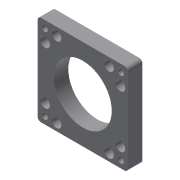
# Autodesk Inventor part: 20_IM_LED_holder
Saved by Autodesk Inventor 2019.4 (Build 234330000, 330)
## iProperties
Created: 2020-10-28
Part Number: 20_IM_LED_holder
Material: Generic
Document SubType Name: Modeling
Designer: wanghaoran
Density: 1 g/cm^3
Appearance: Default
Author: wanghaoran
Autodesk Inventor part; units mm, degrees
ref_plane "YZ Plane" through (0, 0, 0) normal (1, 0, 0) x (0, 1, 0)
ref_plane "XZ Plane" through (0, 0, 0) normal (0, 1, 0) x (-1, 0, 0)
ref_plane "XY Plane" through (0, 0, 0) normal (0, 0, 1) x (1, 0, 0)
sketch "Sketch1" plane through (0, 0, 0) normal (0, 0, 1) x (1, 0, 0)
  line L0 (-25, 25) -> (25, 25)
  line L1 (25, 25) -> (25, -25)
  line L2 (25, -25) -> (-25, -25)
  line L3 (-25, -25) -> (-25, 25)
  line L4 (-25, 25) -> (25, -25) construction
  line L5 (25, 25) -> (-25, -25) construction
  circle A0 centre (0, 0) radius 16
  circle A1 centre (-20.8, -14.5) radius 2.65
  circle A2 centre (-14.5, -20.8) radius 2.65
  circle A3 centre (-20.8, 14.5) radius 2.65
  circle A4 centre (20.8, -14.5) radius 2.65
  circle A5 centre (20.8, 14.5) radius 2.65
  circle A6 centre (-14.5, 20.8) radius 2.65
  circle A7 centre (14.5, -20.8) radius 2.65
  circle A8 centre (14.5, 20.8) radius 2.65
  dimension "d0" = 50
  dimension "d1" = 50
  dimension "d2" = 32
  dimension "d5" = 5.3
  dimension "d6" = 4.2
  dimension "d8" = 10.5
  dimension "d11" = 29
  dimension "d14" = 41.6
  constraints: 12 end point, 9 centre point, 4 symmetric about line, 2 horizontal, 2 midpoint, 2 parallel, 1 coincident, 1 perpendicular, 1 vertical, 10 other
  measures "d0" distance of L1.end L2.end
  measures "d1" distance of L0.end L1.end
  measures "d2" diameter of A0
  measures "d5" diameter of A1
  measures "d6" distance from line of A1.centre L3
  measures "d8" distance from line of L2 A1.centre
  measures "d11" distance of A1.centre A3.centre
  measures "d14" distance of A1.centre A4.centre
extrude "Extrusion1" add sketch "Sketch1" along normal blind 9
fillet "Fillet1" radius 2 4 edges at (-25, 25, 4.5) (25, 25, 4.5) (-25, -25, 4.5) (25, -25, 4.5)
sketch "Sketch2" plane through (0, 0, 9) normal (0, 0, 1) x (1, 0, 0)
  arc A0 (23, -25) -> (25, -23) centre (23, -23) ccw projected
  line L0 (25, -23) -> (25, 23) projected
  arc A1 (25, 23) -> (23, 25) centre (23, 23) ccw projected
  line L1 (23, 25) -> (-23, 25) projected
  arc A2 (-23, 25) -> (-25, 23) centre (-23, 23) ccw projected
  line L2 (-25, 23) -> (-25, -23) projected
  arc A3 (-25, -23) -> (-23, -25) centre (-23, -23) ccw projected
  line L3 (-23, -25) -> (23, -25) projected
  circle A4 centre (14.5, 20.8) radius 2.65 projected
  circle A5 centre (-14.5, 20.8) radius 2.65 projected
  circle A6 centre (14.5, -20.8) radius 2.65 projected
  circle A7 centre (20.8, 14.5) radius 2.65 projected
  circle A8 centre (20.8, -14.5) radius 2.65 projected
  circle A9 centre (-20.8, 14.5) radius 2.65 projected
  circle A10 centre (-14.5, -20.8) radius 2.65 projected
  circle A11 centre (-20.8, -14.5) radius 2.65 projected
  circle A12 centre (0, 0) radius 16 projected
  line L4 (21, -21) -> (-21, -21)
  line L5 (-21, -21) -> (-21, 21)
  line L6 (-21, 21) -> (21, 21)
  line L7 (21, 21) -> (21, -21)
  line L8 (21, -21) -> (-21, 21) construction
  line L9 (-21, -21) -> (21, 21) construction
  circle A13 centre (-28.6, 21.06) radius 1.55 projected
  dimension "d18" = 42
  dimension "d19" = 42
  constraints: 12 end point, 2 midpoint, 2 parallel, 1 horizontal, 1 perpendicular
  measures "d18" distance of L5.end L6.end
  measures "d19" distance of L4.end L5.end
hole "Hole1" at (-21, 21, 9) at (21, 21, 9) at (21, -21, 9) at (-21, -21, 9) direction (0, 0, -1) diameter 3.3 end through all both
body "Solid1"
